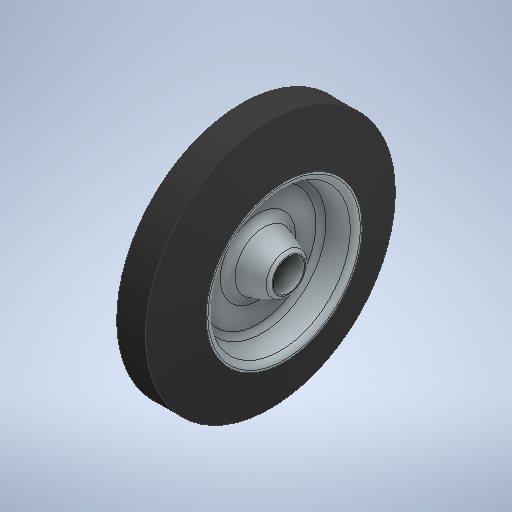
# Autodesk Inventor part: Колесо
Saved by Autodesk Inventor 2025.2 (Build 292293000, 293)
## iProperties
Created: 2025-01-19
Part Number: Колесо
Material: Типовые
Document SubType Name: Modeling
Designer: neket
Density: 1 g/cm^3
Appearance: По умолчанию
Author: neket
Autodesk Inventor part; units mm, degrees
ref_plane "YZ Plane" through (0, 0, 0) normal (1, 0, 0) x (0, 1, 0)
ref_plane "XZ Plane" through (0, 0, 0) normal (0, 1, 0) x (-1, 0, 0)
ref_plane "XY Plane" through (0, 0, 0) normal (0, 0, 1) x (1, 0, 0)
sketch "Эскиз1" plane through (0, 0, 0) normal (0, 0, 1) x (1, 0, 0)
  line L0 (0, 2726.5937) -> (0, -5361.0214)
  line L1 (-7862.4009, 0) -> (14463.6017, 0)
  line L2 (11.5, 100) -> (0, 100)
  line L3 (11.5, 100) -> (22.5, 62.5)
  line L4 (22.5, 62.5) -> (22.5, 61.0236)
  line L5 (1.5, 30.151) -> (1.5, 46.4764)
  line L6 (19.1817, 56.3149) -> (4.8183, 51.1851)
  arc A0 (4.8183, 51.1851) -> (1.5, 46.4764) centre (6.5, 46.4764) ccw
  arc A1 (19.1817, 56.3149) -> (22.5, 61.0236) centre (17.5, 61.0236) ccw
  line L7 (26.218, 12.6167) -> (26.218, 13.4327)
  line L8 (6.3077, 23.1509) -> (24.2949, 16.2327)
  line L9 (26.218, 12.6167) -> (-1.282, 12.6167)
  arc A2 (1.5, 30.151) -> (6.3077, 23.1509) centre (9, 30.151) ccw
  arc A3 (26.218, 13.4327) -> (24.2949, 16.2327) centre (23.218, 13.4327) ccw
  point P0 (0, 0)
  point P1 (0, 12.6167)
  dimension "d32" = 7.5
  dimension "d33" = 3
  constraints: 20 end point, 8 point on circle, 8 tangent, 4 centre point, 2 vertical, 1 equal radius, 1 horizontal
  measures "d32" radius of A2
  measures "d33" radius of A3
revolve "Вращение3" add sketch "Эскиз1" angle 360 about axis through (-7862.4009, 0, 0) along (1, 0, 0)
mirror "Зеркальное отражение5" about plane through (0, 0, 0) normal (1, 0, 0)
